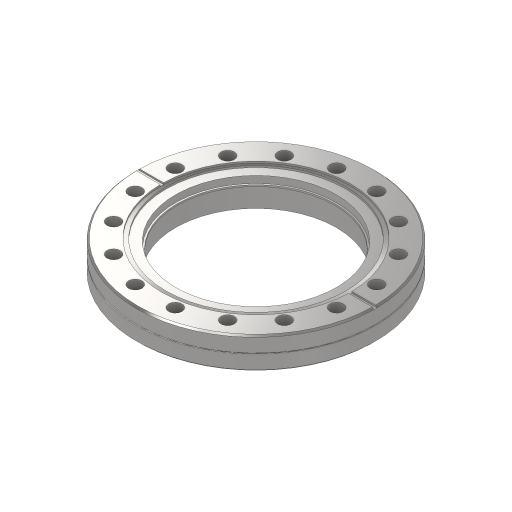
# Autodesk Inventor part: UFC-05
Saved by Autodesk Inventor 2024.2 (Build 282272000, 272)
## iProperties
Created: 2016-09-29
Part Number: UFC-05
Material: Stainless Steel, 440C
Document SubType Name: Modeling
Designer: Arseny
Density: 7.75 g/cm^3
Appearance: Semi-Polished
Mass: 852.704 g
Surface Area: 270.424 cm^2
Volume: 110.026 cm^3
Author: Arseny
Autodesk Inventor part; units mm, degrees
ref_plane "YZ Plane" through (0, 0, 0) normal (1, 0, 0) x (0, 1, 0)
ref_plane "XY Plane" through (0, 0, 0) normal (0, 0, 1) x (1, 0, 0)
sketch "Sketch1" plane through (0, 0, 0) normal (0, 1, 0) x (-1, 0, 0)
  line L0 (-51, -9.9) -> (-75.8, -9.9)
  line L1 (-75.8, -9.9) -> (-75.8, 9.9)
  line L2 (-75.8, 9.9) -> (-59.725, 9.9)
  line L3 (-59.725, 9.9) -> (-59.725, 8.8)
  line L4 (-59.725, 8.8) -> (-57.125, 9.4)
  line L5 (-57.125, 9.4) -> (-57.125, 8.2)
  line L6 (-57.125, 8.2) -> (-51, 8.2)
  line L7 (-51, 3.8) -> (-50, 3.8)
  line L8 (-50, 3.8) -> (-50, 2.8)
  line L9 (-50, 2.8) -> (-51, 2.8)
  line L10 (-51, 2.8) -> (-51, -9.9)
  line L11 (0, 17.0821) -> (0, -17.0821)
  line L12 (0, 0) -> (-89.5532, 0) construction
  line L13 (-51, 8.2) -> (-51, 3.8)
  line L14 (-65.125, 1.8471) -> (-65.125, -11.1229) construction
  point P0 (-75.8, 0)
  dimension "uA" = 151.6
  dimension "uC" = 19.8
  dimension "d4" = 1.1
  dimension "d5" = 0.5
  dimension "d6" = 2.6
  dimension "d7" = 1.7
  dimension "PCD" = 130.25
  dimension "uKnife" = 8
  dimension "uWeld" = 1
  dimension "d13" = 1
  dimension "uK" = 102
  dimension "uB" = 102
  dimension "uD" = 7.1
  constraints: 30 end point, 7 vertical, 6 horizontal, 2 midpoint, 1 coincident, 1 point on line
  measures "uA" diameter of L1 L11
  measures "uC" distance of L0.end L1.end
  measures "d4" distance of L2.end L3.end
  measures "d5" distance from line of L2 L4.end
  measures "d6" distance from line of L3 L4.end
  measures "d7" distance between parallel lines of L2 L6
  measures "PCD" diameter of L14 L11
  measures "uKnife" distance between parallel lines of L5 L14
  measures "uWeld" distance of L7.start L7.end
  measures "d13" distance of L7.end L8.end
  measures "uK" diameter of L13 L11
  measures "uB" diameter of L10 L11
  measures "uD" distance between parallel lines of L9 L2
revolve "Revolution1" add sketch "Sketch1" angle 360 about axis through (0, 0, 17.0821) along (0, 0, -1)
sketch "Sketch2" plane through (0, 0, 9.9) normal (0, 0, 1) x (1, 0, 0)
  line L0 (0, 0) -> (0, 47.8719) construction
  line L1 (0, 0) -> (-12.7053, 63.8736) construction
  circle A0 centre (-12.7053, 63.8736) radius 4.25
  dimension "hole_diam" = 8.5
  dimension "d18" = 65.125
  dimension "bolt_angle" = 11.25
  constraints: 4 end point, 1 centre point, 1 coincident, 1 vertical
  measures "hole_diam" diameter of A0
  measures "d18" distance of L0.start L1.end
  measures "bolt_angle" angle of L0 L1
extrude "Extrusion1" cut sketch "Sketch2" against normal through all
pattern_circular "Circular Pattern1" count 16 over 360 about axis through (0, 0, -10) along (0, 0, 1) of "Extrusion1"
chamfer "Chamfer1" distance 1 angle 45 2 edges at (-75.8, 0, 9.9) (-75.8, 0, -9.9)
sketch "Sketch3" plane through (0, 0, 0) normal (0, 1, 0) x (-1, 0, 0)
  line L0 (-76.3, 0.25) -> (-75.3, 0.25)
  line L1 (-75.3, 0.25) -> (-75.3, -0.25)
  line L2 (-75.3, -0.25) -> (-76.3, -0.25)
  line L3 (-76.3, -0.25) -> (-76.3, 0.25)
  line L4 (0, 0) -> (-75.8, 0) construction
  line L5 (-75.8, -8.9) -> (-75.8, 8.9) construction
  line L6 (-75.3, 0.25) -> (-76.3, -0.25) construction
  line L7 (-76.3, 0.25) -> (-75.3, -0.25) construction
  line L8 (0, -15.82) -> (0, 15.82) projected
  point P0 (-75.3, 0)
  point P1 (-75.8, 0.25)
  dimension "d28" = 1
  dimension "d29" = 0.5
  constraints: 14 end point, 3 midpoint, 3 perpendicular, 2 point on line, 1 coincident, 1 horizontal
  measures "d28" distance of L0.start L0.end
  measures "d29" distance of L0.end L1.end
revolve "Revolution2" cut sketch "Sketch3" angle 360 about axis through (0, 0, -10) along (0, 0, 1)
ref_plane "Work Plane1" through (0, -75.8, 0) normal (0, 1, 0) x (-1, 0, 0)
sketch "Sketch4" plane through (0, -75.8, 0) normal (0, 1, 0) x (-1, 0, 0)
  line L0 (1, 10.9) -> (1, 8.9)
  line L1 (1, 8.9) -> (-1, 8.9)
  line L2 (-1, 8.9) -> (-1, 10.9)
  line L3 (-1, 10.9) -> (1, 10.9)
  line L4 (0, 0) -> (0, 11.6519) construction
  line L5 (-74.8, 9.9) -> (74.8, 9.9) construction
  point P0 (0, 10.9)
  point P1 (-1, 9.9)
  dimension "d31" = 2
  dimension "d32" = 2
  constraints: 10 end point, 3 vertical, 2 midpoint, 2 point on line, 1 horizontal, 1 perpendicular
  measures "d31" distance of L2.end L0.start
  measures "d32" distance of L1.end L2.end
extrude "Extrusion2" cut sketch "Sketch4" along normal up to surface
mirror "Mirror1" about plane through (0, 0, 0) normal (0, 1, 0) of "Extrusion2"
equation "\"d18\" = 0.5 * PCD"
body "Solid1"
